Autodesk Fusion 360 part; units mm, degrees
note: some values were not read from the file. Set by a fixed rule: which face or edge a step refers to.
(part 2 of 2)
sketch "Sketch3" plane through (0, 0, 0) normal (0, 0, 1) x (1, 0, 0)
  circle A0 centre (53.6706, 140.0055) radius 19.7
  circle A1 centre (53.5799, 139.9148) radius 2.95
  circle A2 centre (53.5799, 139.9148) radius 1.55
  circle A3 centre (46.8624, 146.6323) radius 2.95
  circle A4 centre (60.2974, 133.1973) radius 2.95
  line L0 (-45, 67.72) -> (45, 67.72)
  line L1 (39.6502, 153.8445) -> (67.5096, 125.9851) construction
  circle A5 centre (53.6706, 140.0055) radius 21.3
  line L2 (-78.5799, 146.72) -> (-78.5799, 160.72)
  arc A6 (-75, 164.2999) -> (-78.5799, 160.72) centre (-75, 160.72) ccw
  line L3 (-75, 164.2999) -> (-69, 164.2999)
  line L4 (-69, 164.2999) -> (-69, 166.9303)
  line L5 (-69, 166.9303) -> (-67.8, 166.9303)
  line L6 (-67.8, 166.9303) -> (-67.8, 164.2999)
  line L7 (-67.8, 164.2999) -> (-47.2, 164.2999)
  line L8 (-47.2, 164.2999) -> (-47.2, 166.9303)
  line L9 (-47.2, 166.9303) -> (-46, 166.9303)
  line L10 (-46, 166.9303) -> (-46, 164.2999)
  line L11 (-46, 164.2999) -> (46, 164.2999)
  line L12 (46, 164.2999) -> (46, 166.9303)
  line L13 (46, 166.9303) -> (47.2, 166.9303)
  line L14 (47.2, 166.9303) -> (47.2, 164.2999)
  line L15 (47.2, 164.2999) -> (67.8, 164.2999)
  line L16 (67.8, 164.2999) -> (67.8, 166.9303)
  line L17 (67.8, 166.9303) -> (69, 166.9303)
  line L18 (69, 166.9303) -> (69, 164.2999)
  line L19 (69, 164.2999) -> (75, 164.2999)
  arc A7 (78.5799, 160.72) -> (75, 164.2999) centre (75, 160.72) ccw
  line L20 (78.5799, 160.72) -> (78.5799, 146.72)
  line L21 (78.5799, 146.72) -> (81.2103, 146.72)
  line L22 (81.2103, 146.72) -> (81.2103, 143.72)
  line L23 (81.2103, 143.72) -> (78.5799, 143.72)
  line L24 (78.5799, 143.72) -> (78.5799, 87.72)
  line L25 (78.5799, 87.72) -> (81.2103, 87.72)
  line L26 (81.2103, 87.72) -> (81.2103, 84.72)
  line L27 (81.2103, 84.72) -> (78.5799, 84.72)
  line L28 (78.5799, 84.72) -> (78.5799, 70.72)
  arc A8 (75, 67.1401) -> (78.5799, 70.72) centre (75, 70.72) ccw
  line L29 (75, 67.1401) -> (58.1, 67.1401)
  line L30 (58.1, 67.1401) -> (58.1, 64.5097)
  line L31 (58.1, 64.5097) -> (56.9, 64.5097)
  line L32 (56.9, 64.5097) -> (56.9, 67.1401)
  line L33 (56.9, 67.1401) -> (-56.9, 67.1401)
  line L34 (-56.9, 67.1401) -> (-56.9, 64.5097)
  line L35 (-56.9, 64.5097) -> (-58.1, 64.5097)
  line L36 (-58.1, 64.5097) -> (-58.1, 67.1401)
  line L37 (-58.1, 67.1401) -> (-75, 67.1401)
  arc A9 (-78.5799, 70.72) -> (-75, 67.1401) centre (-75, 70.72) ccw
  line L38 (-78.5799, 70.72) -> (-78.5799, 84.72)
  line L39 (-78.5799, 84.72) -> (-81.2103, 84.72)
  line L40 (-81.2103, 84.72) -> (-81.2103, 87.72)
  line L41 (-81.2103, 87.72) -> (-78.5799, 87.72)
  line L42 (-78.5799, 87.72) -> (-78.5799, 143.72)
  line L43 (-78.5799, 143.72) -> (-81.2103, 143.72)
  line L44 (-81.2103, 143.72) -> (-81.2103, 146.72)
  line L45 (-81.2103, 146.72) -> (-78.5799, 146.72)
  line L46 (53.5799, 139.9148) -> (73.3704, 139.9148)
  point P0 (53.6706, 140.0055)
  dimension "d150" = 39.4
  dimension "d152" = 5.9
  dimension "d153" = 3.1
  dimension "d154" = 5.9
  dimension "d155" = 5.9
  dimension "d160" = 19
  dimension "d175" = 9.5
  dimension "d179" = 1.6
  dimension "d330" = 25
  dimension "d331" = 24.3851
  dimension "d332" = 45
  constraint coincident A0 L1.start
  constraint coincident A0 L1.end
  constraint coincident A3.centre L1
  constraint coincident A4.centre L1
  constraint coincident A1.centre L1
  constraint coincident P0 A0.centre
  constraint midpoint A1.centre L1
  constraint coincident A1.centre A2.centre
  constraint coincident A0 L46.end
  constraint horizontal L46
  measures "d150" diameter of A0
  measures "d152" diameter of A1
  measures "d153" diameter of A2
  measures "d154" diameter of A3
  measures "d155" diameter of A4
  measures "d160" distance of A3.centre A4.centre
  measures "d175" distance of A1.centre A3.centre
  measures "d330" distance of A1.centre L24
  measures "d331" distance of A1.centre L11
  measures "d332" angle of L1 L46
extrude "Extrude8" add sketch "Sketch3" along normal blind 8 contours A0 | A1 | A2 | A3 | A4 | A5 sketch seen with x (0, 0, 1) y (1, 0, 0) z (0, 1, 0) at (-115.72, 0, 0) bodies 7 in component "Box Lid"
extrude "Extrude9" cut sketch "Sketch3" along normal blind 5 contours A0 | A1 | A2 | A3 | A4 sketch seen with x (0, 0, 1) y (1, 0, 0) z (0, 1, 0) at (-115.72, 0, 0) bodies 7 in component "Box Lid"
fillet "Fillet8" radius 0.5 1 edges at (17.1617, 0, 35.3037) on bodies 7 in component "Box Lid"
extrude "Extrude2''" cut sketch "Sketch3" along normal blind 10 contours A3 | A4 sketch seen with x (0, 0, 1) y (1, 0, 0) z (0, 1, 0) at (-115.72, 0, 0) bodies 7 in component "Box Lid"
extrude "Extrude3''" cut sketch "Sketch3" along normal through all contours A2 sketch seen with x (0, 0, 1) y (1, 0, 0) z (0, 1, 0) at (-115.72, 0, 0) bodies 7 in component "Box Lid"
fillet "Fillet3''" radius 0.5 3 edges at (29.8456, 5, 44.112) (16.4105, 5, 57.547) (23.6343, 5, 52.1348) on bodies 7 in component "Box Lid"
extrude "Extrude10''" cut sketch "Sketch3" along normal blind 2 from surface at 5 contours A1 | A2 sketch seen with x (0, 0, 1) y (1, 0, 0) z (0, 1, 0) at (-115.72, 0, 0) bodies 7 in component "Box Lid"
fillet "Fillet9" radius 0.5 1 edges at (23.1281, 5, 50.8295) on bodies 7 in component "Box Lid"
sketch "Sketch6 (3)" plane through (82.4, 0, 0) normal (1, 0, 0) x (0, 1, 0)
  line L0 (-27, 3.8201) -> (27, 3.8201)
  line L1 (27, 3.8201) -> (27, 25)
  line L2 (27, 25) -> (-27, 25)
  line L3 (-27, 25) -> (-27, 3.8201)
  circle A0 centre (0, 14.4101) radius 7.55
  line L4 (0, 25) -> (0, 3.8201) construction
  circle A1 centre (0, 14.4101) radius 11.55
  dimension "d202" = 15.1
  dimension "d243" = 4
  constraint midpoint L2 L4.start
  constraint midpoint L0 L4.end
  constraint midpoint A0.centre L4
  measures "d202" diameter of A0
extrude "Extrude1'''" cut sketch "Sketch6 (3)" against normal blind 3 contours A0 sketch seen with x (0, 0, -1) y (-1, 0, 0) z (0, 1, 0) at (0, 0, 0) bodies 2 in component "Box (1)"
fillet "Fillet2''" radius 0.5 2 edges at (7.0391, 17.1402, -82.4) (7.0391, 11.6799, -80) on bodies 2 in component "Box (1)"
sketch "Sketch7 (3)" plane through (0, 0, 0) normal (0, 0, 1) x (1, 0, 0)
extrude "Extrude2'''" cut sketch "Sketch6 (3)" against normal blind 1 contours L0 L2 A1 | L0 A1 | L2 A1 sketch seen with x (0, 0, -1) y (-1, 0, 0) z (0, 1, 0) at (0, 0, 0) bodies 2 in component "Box (1)"
sketch "Sketch8 (3)" plane through (0, 0, 2.4) normal (0, 0, 1) x (-1, 0, 0)
  line L0 (-120.6135, -72.8812) -> (13.4537, -206.9484) construction
  circle A0 centre (-66.6614, -126.8333) radius 2
  circle A1 centre (-40.4984, -152.9963) radius 2
  line L1 (-53.5799, -139.9148) -> (32.2641, -139.9148)
  point P0 (-74.1707, -119.324)
  point P1 (-115.1183, -78.3764)
  point P2 (-74.1707, -119.324)
  point P3 (-115.1183, -78.3764)
  point P4 (-53.5799, -139.9148)
  point P5 (-53.5799, -139.9148)
  dimension "d216" = 4
  dimension "d217" = 4
  dimension "d220" = 18.5
  dimension "d221" = 18.5
  dimension "d329" = 45
  constraint coincident L0 A0.centre
  constraint coincident L0 A1.centre
  constraint coincident L0 P2
  constraint coincident L0 P3
  constraint coincident P2 P0
  constraint coincident P3 P1
  constraint midpoint L0 P5
  constraint coincident P5 P4
  constraint horizontal L1
  measures "d216" diameter of A0
  measures "d217" diameter of A1
  measures "d220" distance of A0.centre P5
  measures "d221" distance of A1.centre P5
  measures "d329" angle of L0 L1
extrude "Extrude5" add sketch "Sketch8 (3)" along normal blind 18 contours A0 sketch seen with x (0, 0, 1) y (1, 0, 0) z (0, 1, 0) at (-115.72, 0, 0) bodies 7 in component "Box Lid"
extrude "Extrude6" add sketch "Sketch8 (3)" along normal blind 18 contours A1 sketch seen with x (0, 0, 1) y (1, 0, 0) z (0, 1, 0) at (-115.72, 0, 0) bodies 7 in component "Box Lid"
fillet "Fillet6" radius 0.5 1 edges at (37.9995, 20.4, 42.3631) on bodies 7 in component "Box Lid"
fillet "Fillet7" radius 0.5 1 edges at (11.8366, 20.4, 68.526) on bodies 7 in component "Box Lid"
sketch "Sketch9 (3)" plane through (-80, 0, 0) normal (1, 0, 0) x (0, 1, 0)
  line L0 (-45, 4.4) -> (45, 4.4)
  line L1 (45, 4.4) -> (45, 32.4)
  line L2 (45, 32.4) -> (-45, 32.4)
  line L3 (-45, 32.4) -> (-45, 4.4)
  circle A0 centre (-21.327, 8.4855) radius 2
  dimension "d238" = 4
  measures "d238" diameter of A0
extrude "Extrude3'''" [suppressed] in component "Box (1)"
fillet "Fillet3'''" [suppressed] in component "Box (1)"
fillet "Fillet4" [suppressed] in component "Box (1)"
sketch "Sketch15" plane through (0, 0, 0) normal (0, 1, 0) x (1, 0, 0) in component "Lid"
  line L0 (97, -30) -> (51, -30)
  line L1 (51, -30) -> (51, -76)
  line L2 (51, -76) -> (97, -76)
  line L3 (97, -76) -> (97, -30)
  line L4 (150, 100) -> (-45.928, 100)
  line L5 (-45.928, 100) -> (-45.928, -138.4961)
  line L6 (-45.928, -138.4961) -> (150, -138.4961)
  line L7 (150, -138.4961) -> (150, 100)
  line L8 (22, 78.5799) -> (78, 78.5799)
  line L9 (95, -78) -> (5, -78)
  dimension "d333" = 2
  constraint horizontal L0
  constraint vertical L1
  constraint horizontal L2
  constraint vertical L3
  constraint horizontal L4
  constraint vertical L5
  constraint horizontal L6
  constraint vertical L7
  measures "d333" distance of L2 L9
extrude "Extrude11''" cut sketch "Sketch3" along normal up to surface (5 mm away) contours A0 sketch seen with x (0, 0, 1) y (1, 0, 0) z (0, 1, 0) at (-115.72, 0, 0) bodies 7 in component "Box Lid"
extrude "Extrude12''" add sketch "Sketch3" along normal blind 4 from surface at 8 contours A1 sketch seen with x (0, 0, 1) y (1, 0, 0) z (0, 1, 0) at (-115.72, 0, 0) bodies 7 in component "Box Lid"
copy_body "CopyPasteBodies1" bodies 7 makes body 10 in component "Box Lid"
extrude "Extrude23" [suppressed] in component "Lid"
extrude "Extrude4" [no effect] in component "Box (1)"
extrude "Extrude1''''" [no effect] in component "Box Latch"
extrude "Extrude7" cut sketch "Sketch15" along normal blind 100 sketch seen with x (1, 0, 0) y (0, 1, 0) z (0, 0, 1) at (-50, 0, 0) bodies 10 in component "Box Lid"
extrude "Extrude2''''" [no effect] in component "Seal"
sketch "Sketch3 (2)" plane through (0, 8, 0) normal (0, 1, 0) x (-1, 0, 0) in component "Box Lid"
  circle A0 centre (-11.1133, 66.6614) radius 2
  circle A1 centre (-17.4773, 60.2974) radius 2.95
  circle A2 centre (-24.1948, 53.5799) radius 2.95
  circle A3 centre (-37.2763, 40.4984) radius 2
  circle A4 centre (-30.9123, 46.8624) radius 2.95
  circle A5 centre (-24.2855, 53.6706) radius 21.3
extrude "Extrude15'" add sketch "Sketch3 (2)" along normal blind 4 bodies 10 in component "Box Lid"
pattern_linear "R-Pattern4" count 2 spacing 48 along (0, 0, -1) count 2 spacing 48 along (-1, 0, 0) of bodies 10 makes body 11 at (26.7666, 12, 14.7148) makes body 12 at (-21.2334, 12, 62.7148) makes body 13 at (-21.2334, 12, 14.7148) in component "Box Lid"
sketch "Sketch1 (5)" plane through (-115.72, 0, 0) normal (0, 1, 0) x (0, 0, 1) in component "Box Lid"
  circle A0 centre (5.6706, 140.0055) radius 21.5
  circle A1 centre (53.6706, 140.0055) radius 21.5
  circle A2 centre (5.6706, 92.0055) radius 21.5
  circle A3 centre (53.6706, 92.0055) radius 21.5
  line L0 (78, 160.72) -> (78, 70.72)
  line L1 (-78, 70.72) -> (-78, 160.72)
  point P0 (53.6706, 140.0055)
  dimension "d297" = 43
  dimension "d301" = 48
  dimension "d302" = -48
  constraint coincident P0 A1.centre
  measures "d297" diameter of A0
extrude "Extrude13''" cut sketch "Sketch1 (5)" along normal blind 50 bodies 7 in component "Box Lid"
sketch "Sketch16" plane through (0, 2.4, 0) normal (0, 1, 0) x (-1, 0, 0) in component "Lid"
  circle A0 centre (-74.2855, 53.6706) radius 21.5
  circle A1 centre (-26.2855, 53.6706) radius 21.5
  circle A2 centre (-74.2855, 5.6706) radius 21.5
  circle A3 centre (-26.2855, 5.6706) radius 21.5
  arc A4 (-5, -78) -> (-2, -75) centre (-5, -75) ccw
  line L0 (-2, -75) -> (-2, 75)
  arc A5 (-2, 75) -> (-5, 78) centre (-5, 75) ccw
  line L1 (-5, 78) -> (-95, 78)
  arc A6 (-95, 78) -> (-98, 75) centre (-95, 75) ccw
  line L2 (-98, 75) -> (-98, -75)
  arc A7 (-98, -75) -> (-95, -78) centre (-95, -75) ccw
  line L3 (-95, -78) -> (-5, -78)
  circle A8 centre (-12, -72) radius 1.75
  circle A9 centre (-44.5, -72) radius 1.75
  circle A10 centre (-12, -28.5) radius 1.75
  circle A11 centre (-44.5, -28.5) radius 1.75
  circle A12 centre (-12, -72) radius 3.75
  circle A13 centre (-44.5, -72) radius 3.75
  circle A14 centre (-44.5, -28.5) radius 3.75
  circle A15 centre (-12, -28.5) radius 3.75
  line L4 (-49, -18) -> (-3, -18)
  circle A16 centre (-55.5, -72) radius 3.75
  circle A17 centre (-55.5, -72) radius 1.75
  circle A18 centre (-55.5, -28.5) radius 3.75
  circle A19 centre (-55.5, -28.5) radius 1.75
  circle A20 centre (-88, -28.5) radius 1.75
  circle A21 centre (-88, -28.5) radius 3.75
  circle A22 centre (-88, -72) radius 3.75
  circle A23 centre (-88, -72) radius 1.75
  point P0 (-44.5, -72)
  point P1 (-12, -28.5)
  point P2 (-44.5, -28.5)
  dimension "d313" = 3.5
  dimension "d314" = 32.5
  dimension "d315" = 3.5
  dimension "d316" = 3.5
  dimension "d317" = 43.5
  dimension "d318" = 3.5
  dimension "d319" = 43.5
  dimension "d334" = 6
  dimension "d335" = 2
  dimension "d336" = 2
  dimension "d337" = 2
  dimension "d338" = 2
  dimension "d352" = 6
  dimension "d354" = 10
  dimension "d357" = 2
  dimension "d358" = 2
  dimension "d359" = 2
  dimension "d360" = 2
  dimension "d361" = 3.5
  dimension "d362" = 3.5
  dimension "d363" = 3.5
  dimension "d364" = 43.5
  dimension "d365" = 3.5
  dimension "d368" = 32.5
  dimension "d369" = 10
  dimension "d371" = 11
  constraint coincident P0 A9.centre
  constraint coincident P1 A10.centre
  constraint coincident P2 A11.centre
  constraint horizontal P1 P2
  constraint vertical A8.centre P1
  constraint vertical A16.centre A18.centre
  constraint horizontal A16.centre A22.centre
  constraint horizontal A20.centre A18.centre
  constraint vertical A20.centre A22.centre
  measures "d313" diameter of A8
  measures "d314" distance of A8.centre P0
  measures "d315" diameter of A9
  measures "d316" diameter of A10
  measures "d317" distance of A8.centre P1
  measures "d318" diameter of A11
  measures "d319" distance of P0 P2
  measures "d334" distance of L3 A8.centre
  measures "d352" distance of L3 P0
  measures "d354" distance of L0 A8.centre
  measures "d361" diameter of A17
  measures "d362" diameter of A23
  measures "d363" diameter of A19
  measures "d364" distance of A16.centre A18.centre
  measures "d365" diameter of A20
  measures "d368" distance of A16.centre A22.centre
  measures "d369" distance of L2 A22.centre
  measures "d371" distance of P2 A18.centre
extrude "Extrude17'" add sketch "Sketch16" along normal blind 6.5 separate body contours A12 | A13 | A14 | A15 | A16 | A18 | A21 | A22 sketch seen with x (1, 0, 0) y (0, 1, 0) z (0, 0, 1) at (-50, 0, 0) makes body 14 at (41.6756, 6.7333, -71.257) makes body 15 at (-9.134, 6.7333, -71.0747) makes body 16 at (-41.7453, 6.7333, -28.6869) makes body 17 at (34.2547, 6.7333, -28.6869) makes body 18 at (1.866, 6.7333, -71.0747) makes body 19 at (-41.634, 6.7333, -71.0747) makes body 20 at (-9.2453, 6.7333, -28.6869) makes body 21 at (1.7547, 6.7333, -28.6869) in component "Box Lid"
sketch "Sketch17" plane through (0, 2.4, 0) normal (0, 1, 0) x (-1, 0, 0) in component "Lid"
  circle A0 centre (-74.2855, 53.6706) radius 21.5
  circle A1 centre (-26.2855, 53.6706) radius 21.5
  circle A2 centre (-74.2855, 5.6706) radius 21.5
  circle A3 centre (-26.2855, 5.6706) radius 21.5
  arc A4 (-5, -78) -> (-2, -75) centre (-5, -75) ccw
  line L0 (-2, -75) -> (-2, 75)
  arc A5 (-2, 75) -> (-5, 78) centre (-5, 75) ccw
  line L1 (-5, 78) -> (-95, 78)
  arc A6 (-95, 78) -> (-98, 75) centre (-95, 75) ccw
  line L2 (-98, 75) -> (-98, -75)
  arc A7 (-98, -75) -> (-95, -78) centre (-95, -75) ccw
  line L3 (-95, -78) -> (-5, -78)
  circle A8 centre (-25.6615, -58) radius 1.5
  circle A9 centre (-42.1615, -58) radius 1.5
  circle A10 centre (-58.6615, -58) radius 1.5
  circle A11 centre (-75.1615, -58) radius 1.5
  dimension "d340" = 3
  dimension "d345" = 16.5
  dimension "d346" = 0
  dimension "d348" = 20
  measures "d340" diameter of A8
  measures "d348" distance of L3 A8.centre
extrude "Extrude18'" cut sketch "Sketch17" against normal through all contours A8 | A9 | A10 | A11 sketch seen with x (1, 0, 0) y (0, 1, 0) z (0, 0, 1) at (-50, 0, 0) bodies 7 in component "Box Lid"
sketch "Sketch11" plane through (0, 0, 80) normal (0, 0, -1) x (1, 0, 0) in component "Box"
  line L0 (45, -4.4) -> (-45, -4.4)
  line L1 (-45, -4.4) -> (-45, -32.4)
  line L2 (-45, -32.4) -> (45, -32.4)
  line L3 (45, -32.4) -> (45, -4.4)
  circle A0 centre (0.0249, -14.45) radius 7.55
  dimension "d349" = 15.1
  measures "d349" diameter of A0
extrude "Extrude5'" cut sketch "Sketch11" against normal up to surface (2.4 mm away) contours A0 bodies 2 in component "Box (1)"
fillet "Fillet1" [suppressed] in component "Box (1)"
component "Box" placed x (0, -1, 0) y (0, 0, 1) z (-1, 0, 0) at (0, 0, 0)
component "Lid" placed x (0, 1, 0) y (0, 0, 1) z (1, 0, 0) at (0, 65.72, 0)
component "Seal" placed x (1, 0, 0) y (0, 1, 0) z (0, 0, 1) at (0, 0, 0)
component "Box (1)" placed x (1, 0, 0) y (0, 1, 0) z (0, 0, 1) at (0, 0, 0) in component "Box"
component "Box Latch" placed x (1, 0, 0) y (0, -1, 0) z (0, 0, -1) at (-324.9667, 84.4068, 66.6) in component "Box"
component "Box Lid" placed x (1, 0, 0) y (0, 1, 0) z (0, 0, 1) at (50, 0, 0) in component "Lid"
component "Box Lid" placed x (1, 0, 0) y (0, 1, 0) z (0, 0, 1) at (50, 0, 0) in component "Lid"
equation "InnerBoxDepth = 100 mm" comment "Inner depth"
equation "InnerBoxWidth = 160 mm" comment "Inner width"
equation "InnerBoxBottomHeight = 30 mm" comment "Inner height of the bottom part"
equation "d6 = InnerBoxWidth - 2 * InnerChamferSize"
equation "d7 = InnerBoxDepth - 2 * InnerChamferSize"
equation "d9 = InnerCornerRadius"
equation "d12 = InnerBoxDepth / 2 - InnerChamferSize"
equation "d13 = WallThickness"
equation "d26 = WallThickness"
equation "d27 = InnerChamferSize"
equation "d28 = InnerChamferSize"
equation "d29 = InnerBoxBottomHeight + WallThickness"
equation "d31 = WallThickness"
equation "d46 = RibOffset - InnerBoxDepth / 2"
equation "d47 = InnerBoxWidth / 2 - InnerChamferSize"
equation "d48 = WallThickness"
equation "d49 = InnerChamferSize"
equation "d50 = InnerChamferSize"
equation "d53 = d52"
equation "d54 = RibWidth"
equation "d56 = InnerBoxBottomHeight - 3 mm + WallThickness"
equation "d57 = InnerBoxDepth / 2 - RibOffset"
equation "d58 = -RibWidth"
equation "d60 = HingeLatchOffset - InnerBoxWidth / 2"
equation "d63 = ScrewDiameter + HingeLatchHolesTolerance"
equation "d64 = LatchDistance / 2"
equation "d68 = ScrewLength"
equation "d71 = -( HingeLatchOffset - InnerBoxWidth / 2 )"
equation "d72 = -ScrewLength"
equation "d81 = HingeLatchRibWidth"
equation "d83 = -HingeLatchRibWidth"
equation "d85 = -HingeLatchRibWidth"
equation "d87 = HingeLatchRibWidth"
equation "d98 = ScrewDiameter + 0.2 mm"
equation "d100 = LatchDistance"
equation "d101 = ScrewDiameter + 0.2 mm"
equation "d105 = ScrewDiameter + 0.2 mm"
equation "d108 = ( ScrewLength - 2 * HingeLatchRibWidth ) - LatchWidthTolerance"
equation "ScrewDiameter = 3 mm" comment "M3 => 3 mm"
equation "InnerCornerRadius = 3 mm" comment "Corner radius on the bottom (bottom of champfer)"
equation "HingeLatchOffset = 10 mm" comment "Offset of the hinge and latch from inner wall"
equation "d131 = WallThickness"
equation "WallThickness = 2.4 mm" comment "Thickness of the walls"
equation "RibWidth = 5 mm" comment "Width of the ribs on the sides"
equation "d137 = ScrewDiameter + HingeLatchHolesTolerance"
equation "d138 = HingeOuterDiameter / 2 + 0.2 mm"
equation "d139 = HingeOuterDiameter"
equation "d141 = HingeLatchRibWidth + HingeOuterExtend"
equation "d143 = -HingeLatchRibWidth - HingeOuterExtend"
equation "d145 = -HingeLatchRibWidth - HingeOuterExtend"
equation "d147 = HingeLatchRibWidth + HingeOuterExtend"
equation "InnerChamferSize = 2 mm" comment "Size of the chamfer on the top and bottom inside the box"
equation "d6_1 = InnerBoxWidth - 2 * InnerChamferSize"
equation "d7_1 = InnerBoxDepth - 2 * InnerChamferSize"
equation "d9_1 = InnerCornerRadius"
equation "d12_1 = InnerBoxDepth / 2 - InnerChamferSize"
equation "d13_1 = WallThickness"
equation "d26_1 = WallThickness"
equation "d27_1 = InnerChamferSize"
equation "d28_1 = InnerChamferSize"
equation "d29_1 = InnerBoxLidHeight + WallThickness"
equation "d31_1 = WallThickness"
equation "d46_1 = RibOffset - InnerBoxDepth / 2"
equation "d47_1 = InnerBoxWidth / 2 - InnerChamferSize"
equation "d48_1 = WallThickness"
equation "d49_1 = InnerChamferSize"
equation "d50_1 = InnerChamferSize"
equation "d53_1 = d52_1"
equation "d54_1 = RibWidth"
equation "d56_1 = InnerBoxLidHeight - 3 mm + WallThickness"
equation "d57_1 = InnerBoxDepth / 2 - RibOffset"
equation "d58_1 = -RibWidth"
equation "d60_1 = HingeLatchOffset - InnerBoxWidth / 2"
equation "d63_1 = ScrewDiameter + HingeLatchHolesTolerance"
equation "d64_1 = LatchDistance / 2"
equation "d68_1 = ScrewLength"
equation "d71_1 = -( HingeLatchOffset - InnerBoxWidth / 2 )"
equation "d72_1 = -ScrewLength"
equation "d81_1 = HingeLatchRibWidth"
equation "d83_1 = -HingeLatchRibWidth"
equation "d85_1 = -HingeLatchRibWidth"
equation "d87_1 = HingeLatchRibWidth"
equation "d134 = WallThickness"
equation "d156 = ScrewDiameter + HingeLatchHolesTolerance"
equation "d157 = HingeOuterDiameter / 2 + 0.2 mm"
equation "d158 = HingeOuterDiameter"
equation "d162 = HingeLatchOffset - InnerBoxWidth / 2 + ScrewLength / 2"
equation "d163 = ( ScrewLength - 2 * HingeLatchRibWidth - HingeWidthTolerance - HingeOuterExtend * 2 ) / 2"
equation "d165 = InnerBoxWidth / 2 - HingeLatchOffset - ScrewLength / 2"
equation "d166 = ( ScrewLength - 2 * HingeLatchRibWidth - HingeWidthTolerance - HingeOuterExtend * 2 ) / 2"
equation "d168 = HingeLatchRibWidth / 2"
equation "d170 = HingeLatchRibWidth / 2"
equation "ScrewThreadDiameter = ScrewDiameter - 0.15 mm" comment "Diameter of the inner holes where you screw in the screw"
equation "ScrewLength = 25 mm" comment "Length of the screw to use"
equation "HingeWidthTolerance = 0.25 mm" comment "Tolerance of the hinge (width)"
equation "d24 = ScrewThreadDiameter"
equation "d25 = ScrewThreadDiameter"
equation "d39 = ScrewThreadDiameter"
equation "d40 = ScrewThreadDiameter"
equation "d41 = ScrewThreadDiameter"
equation "d42 = ScrewThreadDiameter"
equation "d51 = HingeWidthTolerance / 2"
equation "RibOffset = 18 mm" comment "Offset of the ribs from inner wall"
equation "LatchDistance = 16 mm" comment "Distance between the two screws of the latch"
equation "InnerBoxLidHeight = 30 mm" comment "Inner height of the lid"
equation "HingeLatchHolesTolerance = 0.4 mm" comment "Tolerance of the hinge and latch holes"
equation "LatchWidthTolerance = 0.4 mm" comment "Tollerance of the latch width"
equation "d89 = SealHeight"
equation "SealHeight = 1.4 mm" comment "Height of the seal"
equation "d97 = LatchWidthTolerance / 2"
equation "HingeLatchRibWidth = 3.2 mm" comment "Width of the ribs for the hinges and latches"
equation "d111 = d113"
equation "d114 = BoxLatchRibChamferOffset"
equation "d117 = d116"
equation "d118 = LidLatchRibChamferOffset"
equation "BoxLatchRibChamferOffset = 17 mm" comment "Offset of the big chamfer on the rib of the box (bottom part).  You can use it to make the latch easier to open (by decreasing it) or make it more protected (by increasing it)"
equation "HingeRibChamferOffset = 5 mm" comment "Offset of the big chamfer on the rib of the hinge side"
equation "HingeOuterDiameter = 6.8 mm" comment "Outer diameter of the hinge.  You can increase it to make it more sturdy (would not recommend to increase it too much)"
equation "d123 = HingeRibChamferOffset"
equation "LidLatchRibChamferOffset = 10 mm" comment "Offset of the big chamfer on the rib of the lid"
equation "d125 = HingeRibChamferOffset"
equation "HingeOuterExtend = 3 mm" comment "How much the outer parts of the hinge should be extended.  Will make it more sturdy and less prone to break.  Should only be increased when using a screw >=30mm"
named bodies: "Box Waterproof", "Latch", "Box - Latch", "Box - Bottom", "Box - Lid", "Box - Seal", "Box - Latch (1)", "Box - Socket", "Box - Socket (1)", "Box - Socket (2)", "Box - Socket (3)"
